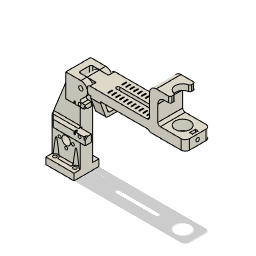
Pen-holder (Autodesk Fusion 360 design; units mm, degrees)
Autodesk Fusion 360 part; units mm, degrees
note: some values were not read from the file. Chosen so that the rebuilt part matches the saved one: which face or edge a step refers to; which pieces of a blend or face edit are solid. Set by a fixed rule: which sketch regions a step uses.
(part 1 of 2)
sketch "Sketch2" plane through (0, 0, 0) normal (0, 1, 0) x (1, 0, 0)
  circle A0 centre (1.8589, 40.0895) radius 2.1
  circle A1 centre (25.8589, 22.0895) radius 2.1
  circle A2 centre (25.8589, 40.0895) radius 2.1
  line L0 (-3.1411, 46.0895) -> (30.8589, 46.0895)
  line L1 (1.8589, 40.0895) -> (25.8589, 22.0895) construction
  line L2 (30.8589, 16.0895) -> (-3.1411, 16.0895)
  line L3 (30.8589, 46.0895) -> (30.8589, 16.0895)
  line L4 (-3.1411, 16.0895) -> (-3.1411, 46.0895)
  line L5 (25.8589, 40.0895) -> (1.8589, 22.0895) construction
  circle A3 centre (1.8589, 22.0895) radius 2.1
  point P0 (13.8589, 31.0895)
  dimension "d22" = 30
  dimension "d24" = 18
  dimension "d25" = 18
  dimension "d26" = 4.2
  dimension "d27" = 4.2
  dimension "d28" = 4.2
  dimension "d29" = 4.2
  dimension "d30" = 15
  dimension "d453" = 18
  dimension "d617" = 17
  dimension "d618" = 34
  constraint horizontal L0
  constraint vertical L3
  constraint horizontal L2
  constraint vertical L4
  constraint coincident A0.centre L1.start
  constraint coincident A1.centre L1.end
  constraint coincident A2.centre L5.start
  constraint coincident L5.end A3.centre
  constraint midpoint P0 L1
  measures "d22" distance of L0 L2
  measures "d24" distance of A2.centre A1.centre
  measures "d25" distance of L5.end A0.centre
  measures "d26" diameter of A0
  measures "d27" diameter of A2
  measures "d28" diameter of A1
  measures "d29" diameter of A3
  measures "d30" distance of P0 L2
  measures "d453" vertical distance of A1.centre A0.centre
  measures "d617" distance of P0 L3
  measures "d618" distance of L0.start L0.end
extrude "Extrude2" add sketch "Sketch2" along normal blind 8 makes body 1
sketch "Sketch3" plane through (0, 8, 0) normal (0, 1, 0) x (-1, 0, 0)
  circle A0 centre (-1.8589, -22.0895) radius 2.1
  circle A1 centre (-25.8589, -22.0895) radius 2.1
  circle A2 centre (-1.8589, -40.0895) radius 2.1
  circle A3 centre (-25.8589, -40.0895) radius 2.1
  line L0 (3.1411, -16.0895) -> (-30.8589, -16.0895)
  line L1 (-30.8589, -16.0895) -> (-30.8589, -46.0895)
  line L2 (-30.8589, -46.0895) -> (3.1411, -46.0895)
  line L3 (3.1411, -46.0895) -> (3.1411, -16.0895)
  line L4 (3.1411, -38.5895) -> (-30.8589, -38.5895)
  line L5 (-30.8589, -38.5895) -> (-30.8589, -23.5895)
  line L6 (-30.8589, -23.5895) -> (3.1411, -23.5895)
  line L7 (3.1411, -23.5895) -> (3.1411, -38.5895)
  circle A4 centre (-1.8589, -40.0895) radius 3.5
  circle A5 centre (-25.8589, -40.0895) radius 3.5
  circle A6 centre (-25.8589, -22.0895) radius 3.5
  circle A7 centre (-1.8589, -22.0895) radius 3.5
  dimension "d46" = 15
  dimension "d47" = 1.5
  dimension "d48" = 18
  dimension "d49" = 7
  dimension "d50" = 7
  dimension "d51" = 7
  dimension "d52" = 7
  constraint horizontal L4
  constraint vertical L5
  constraint horizontal L6
  constraint vertical L7
  constraint coincident L1 L5.end
  constraint coincident L3 L4.start
  constraint concentric A2 A4
  constraint concentric A3 A5
  constraint concentric A1 A6
  constraint concentric A0 A7
  measures "d46" distance of L4 L6
  measures "d47" distance of A2.centre L4
  measures "d48" distance of A0.centre A2.centre
  measures "d49" diameter of A7
  measures "d50" diameter of A6
  measures "d51" diameter of A5
  measures "d52" diameter of A4
extrude "Extrude3" add sketch "Sketch3" along normal blind 41 contours A0 L6 | A0 L6 A7 | L1 L3 L4 L5 L6 L7 A4 A5 A6 A7 | A1 L6 A6 | A1 L6 | A2 L4 A4 | A2 L4 | A3 L4 A5 | A3 L4 picked at (-2.2737, -23.6533) picked at (-1.6456, -25.1095) picked at (-26.0721, -25.1095) picked at (-26.2737, -23.6533) picked at (-2.0721, -37.0694) picked at (-1.9915, -38.2108) picked at (-25.6456, -37.0694) picked at (-25.8096, -38.3912) bodies 1
sketch "Sketch4" plane through (0, 0, -38.5895) normal (0, 0, -1) x (-1, 0, 0)
  line L0 (-0.3892, 8) -> (3.1411, 8)
  line L1 (3.1411, 8) -> (3.1411, 49)
  line L2 (3.1411, 49) -> (-30.8589, 49)
  line L3 (-30.8589, 49) -> (-30.8589, 8)
  circle A0 centre (-13.8589, 30) radius 11.1
  circle A1 centre (-13.8589, 30) radius 5.2
  line L4 (3.1411, 0) -> (-30.8589, 0)
  line L5 (-30.8589, 8) -> (-27.3286, 8)
  line L6 (-27.3286, 8) -> (-24.3892, 8)
  line L7 (-24.3892, 8) -> (-3.3286, 8)
  line L8 (-3.3286, 8) -> (-0.3892, 8)
  dimension "d40" = 10.4
  dimension "d41" = 22.2
  dimension "d66" = 30
  dimension "d619" = 34
  dimension "d620" = 17
  dimension "d621" = 17
  measures "d40" diameter of A1
  measures "d41" diameter of A0
  measures "d66" distance of A0.centre L4
  measures "d619" distance of L1.end L2.end
  measures "d620" distance of L3 A0.centre
  measures "d621" distance of L3 A0.centre
extrude "Extrude4" cut sketch "Sketch4" against normal blind 5 contours A0 bodies 1
extrude "Extrude5" cut sketch "Sketch4" against normal blind 15 contours A1 bodies 1
sketch "Sketch6" plane through (0, 0, -33.5895) normal (0, 0, -1) x (-1, 0, 0)
  circle A0 centre (-13.8589, 30) radius 5.2
  line L0 (-13.8589, 30) -> (10.0526, 30) construction
  line L1 (-13.8589, 30) -> (-13.8589, 48.2161) construction
  line L2 (-13.8589, 30) -> (-31.0155, 30) construction
  line L3 (-13.8589, 30) -> (-13.8589, 12.744) construction
  circle A1 centre (-13.8589, 30) radius 8 construction
  circle A2 centre (-13.8589, 38) radius 1.75
  circle A3 centre (-5.8589, 30) radius 1.75
  circle A4 centre (-13.8589, 22) radius 1.75
  circle A5 centre (-21.8589, 30) radius 1.75
  circle A6 centre (-13.8589, 30) radius 11.1
  dimension "d60" = 16
  dimension "d61" = 3.5
  dimension "d62" = 3.5
  dimension "d63" = 3.5
  dimension "d64" = 3.5
  constraint coincident A0.centre L0.start
  constraint horizontal L0
  constraint perpendicular L0 L1
  constraint perpendicular L1 L2
  constraint perpendicular L0 L3
  constraint coincident A1 A2.centre
  constraint coincident L1 A2.centre
  constraint coincident L0 A3.centre
  constraint coincident A1 A3.centre
  constraint coincident A1 A4.centre
  constraint coincident L3 A4.centre
  constraint coincident A1 A5.centre
  constraint coincident L2 A5.centre
  measures "d60" diameter of A1
  measures "d61" diameter of A2
  measures "d62" diameter of A5
  measures "d63" diameter of A4
  measures "d64" diameter of A3
extrude "Extrude8" cut sketch "Sketch6" against normal through all contours A2 | A3 | A4 | A5 bodies 1
sketch "Sketch7" plane through (0, 0, -38.5895) normal (0, 0, -1) x (-1, 0, 0)
  line L0 (3.1411, 8) -> (3.1411, 49)
  line L1 (3.1411, 49) -> (-30.8589, 49)
  line L2 (-30.8589, 49) -> (-30.8589, 8)
  line L3 (-30.8589, 49) -> (-20.8589, 49)
  line L4 (-20.8589, 49) -> (-20.8589, 109)
  line L5 (-20.8589, 109) -> (-30.8589, 109)
  line L6 (-30.8589, 109) -> (-30.8589, 49)
  line L7 (3.1411, 49) -> (-20.8589, 109)
  line L8 (-30.8589, 109) -> (-6.8589, 49)
  line L9 (-30.8589, 8) -> (-27.3286, 8)
  line L10 (-27.3286, 8) -> (-24.3892, 8)
  line L11 (-24.3892, 8) -> (-3.3286, 8)
  line L12 (-3.3286, 8) -> (-0.3892, 8)
  line L13 (-0.3892, 8) -> (3.1411, 8)
  circle A0 centre (-13.8589, 30) radius 11.1
  line L14 (-30.8589, 109) -> (3.1411, 109)
  line L15 (3.1411, 109) -> (3.1411, 99)
  line L16 (3.1411, 99) -> (-30.8589, 99)
  line L17 (-30.8589, 99) -> (-30.8589, 109)
  line L18 (3.1411, 49) -> (-6.8589, 49)
  line L19 (-6.8589, 49) -> (-6.8589, 109)
  line L20 (-6.8589, 109) -> (3.1411, 109)
  line L21 (3.1411, 109) -> (3.1411, 49)
  dimension "d72" = 60
  dimension "d73" = 10
  dimension "d639" = 10
  dimension "d640" = 10
  dimension "d641" = 10
  constraint horizontal L3
  constraint vertical L4
  constraint horizontal L5
  constraint vertical L6
  constraint coincident L1.end L2.start
  constraint coincident L0.end L1.start
  constraint coincident L1 L8.end
  constraint parallel L7 L8
  constraint horizontal L14
  constraint vertical L15
  constraint horizontal L16
  constraint vertical L17
  constraint horizontal L18
  constraint vertical L19
  constraint horizontal L20
  constraint vertical L21
  constraint coincident L14 L19.end
  measures "d72" distance of L3 L5
  measures "d73" distance of L4 L6
  measures "d639" distance of L19 L21
  measures "d640" distance of L14.end L15.end
  measures "d641" distance of L14.end L19
extrude "Extrude9" add sketch "Sketch7" against normal up to surface (15 mm away) contours L1 L7 L18 L19 | L1 L4 L8 | L4 L7 L8 L16 L19 | L1 L3 L4 L6 L8 L16 | L4 L8 L16 | L4 L7 L16 | L4 L5 L8 L14 L16 | L6 L8 L16 L17 bodies 1
sketch "Sketch8" plane through (0, 0, -23.5895) normal (0, 0, 1) x (1, 0, 0)
  line L0 (-3.1411, 49) -> (-3.1411, 8)
  line L1 (30.8589, 8) -> (30.8589, 109)
  line L2 (30.8589, 109) -> (20.8589, 109)
  circle A0 centre (5.8589, 30) radius 1.75
  circle A1 centre (13.8589, 22) radius 1.75
  line L3 (30.8589, 85.9) -> (44.3589, 85.9)
  line L4 (44.3589, 85.9) -> (44.3589, 80.9)
  line L5 (44.3589, 80.9) -> (30.8589, 80.9)
  line L6 (30.8589, 80.9) -> (30.8589, 85.9)
  line L7 (30.8589, 46.9) -> (44.3589, 46.9)
  line L8 (44.3589, 46.9) -> (44.3589, 51.9)
  line L9 (44.3589, 51.9) -> (30.8589, 51.9)
  line L10 (30.8589, 51.9) -> (30.8589, 46.9)
  circle A2 centre (39.1589, 100.9) radius 8.1
  circle A3 centre (39.1589, 100.9) radius 5.1
  line L11 (39.1589, 100.9) -> (39.1589, 102.6668) construction
  line L12 (39.1589, 100.9) -> (39.1589, 81) construction
  line L13 (39.1589, 109) -> (30.8589, 109)
  line L14 (39.1589, 92.8) -> (30.8589, 92.8)
  line L15 (39.1589, 100.9) -> (49.3712, 90.6877) construction
  line L16 (39.1589, 100.9) -> (45.8085, 100.9) construction
  line L17 (44.8864, 95.1724) -> (30.8589, 81.1449)
  circle A4 centre (37.6089, 49.4) radius 1.75
  circle A5 centre (37.6089, 83.4) radius 1.75
  circle A6 centre (39.1589, 100.9) radius 2.6
  line L18 (20.8589, 109) -> (30.8589, 109)
  line L19 (30.8589, 109) -> (30.8589, 81.1449)
  line L20 (30.8589, 81.1449) -> (20.8589, 81.1449)
  line L21 (20.8589, 81.1449) -> (20.8589, 109)
  line L22 (30.8589, 46.9) -> (20.8589, 46.9)
  line L23 (20.8589, 46.9) -> (20.8589, 51.9)
  line L24 (20.8589, 51.9) -> (30.8589, 51.9)
  line L25 (30.8589, 51.9) -> (30.8589, 46.9)
  line L26 (30.8589, 85.9) -> (20.8589, 85.9)
  line L27 (20.8589, 85.9) -> (20.8589, 80.9)
  line L28 (20.8589, 80.9) -> (30.8589, 80.9)
  line L29 (30.8589, 80.9) -> (30.8589, 85.9)
  line L30 (20.8589, 46.9) -> (44.3589, 46.9)
  line L31 (44.3589, 46.9) -> (44.3589, 51.6551)
  line L32 (44.3589, 51.6551) -> (20.8589, 51.6551)
  line L33 (20.8589, 51.6551) -> (20.8589, 46.9)
  line L34 (44.3589, 85.9) -> (20.8589, 85.9)
  line L35 (20.8589, 85.9) -> (20.8589, 81.1449)
  line L36 (20.8589, 81.1449) -> (44.3589, 81.1449)
  line L37 (44.3589, 81.1449) -> (44.3589, 85.9)
  line L38 (-3.1411, 8) -> (0.3892, 8)
  circle A7 centre (13.8589, 38) radius 1.75
  circle A8 centre (21.8589, 30) radius 1.75
  circle A9 centre (13.8589, 30) radius 5.2
  line L39 (0.3892, 8) -> (3.3286, 8)
  line L40 (3.3286, 8) -> (24.3892, 8)
  line L41 (24.3892, 8) -> (27.3286, 8)
  line L42 (27.3286, 8) -> (30.8589, 8)
  line L43 (20.8589, 109) -> (19.6589, 109)
  line L44 (19.6589, 109) -> (19.6589, 81)
  line L45 (19.6589, 81) -> (20.8589, 81)
  line L46 (20.8589, 81) -> (20.8589, 109)
  line L47 (20.8589, 51.9) -> (5.8589, 51.9)
  line L48 (5.8589, 51.9) -> (5.8589, 46.9)
  line L49 (5.8589, 46.9) -> (20.8589, 46.9)
  line L50 (20.8589, 46.9) -> (20.8589, 51.9)
  line L51 (5.8589, 46.9) -> (44.3589, 46.9)
  line L52 (44.3589, 46.9) -> (44.3589, 43.4)
  line L53 (44.3589, 43.4) -> (5.8589, 43.4)
  line L54 (5.8589, 43.4) -> (5.8589, 46.9)
  line L55 (20.8589, 109) -> (-3.1411, 49)
  dimension "d76" = 29
  dimension "d77" = 13.5
  dimension "d78" = 13.5
  dimension "d79" = 5
  dimension "d80" = 5
  dimension "d81" = 10.2
  dimension "d84" = 16.2
  dimension "d85" = 16.2
  dimension "d86" = 8.3
  dimension "d87" = 45
  dimension "d90" = 3.5
  dimension "d91" = 3.5
  dimension "d92" = 2.5
  dimension "d93" = 2.5
  dimension "d94" = 6.75
  dimension "d95" = 6.75
  dimension "d100" = 5.2
  dimension "d101" = 15
  dimension "d117" = 5
  dimension "d118" = 5
  dimension "d119" = 10
  dimension "d121" = 10
  dimension "d124" = 23.5
  dimension "d125" = -4.7551
  dimension "d126" = -4.7551
  dimension "d642" = 10
  dimension "d643" = 23.1
  dimension "d644" = 23.1
  dimension "d646" = 5
  dimension "d662" = 3.5
  constraint horizontal L3
  constraint vertical L4
  constraint horizontal L5
  constraint vertical L6
  constraint coincident L1 L3.start
  constraint horizontal L7
  constraint vertical L8
  constraint horizontal L9
  constraint vertical L10
  constraint coincident L1 L7.start
  constraint concentric A2 A3
  constraint coincident A2.centre A3.centre
  constraint vertical L11
  constraint parallel L11 L12
  constraint coincident A2 L13.start
  constraint coincident L11 L13.start
  constraint coincident L1 L2.start
  constraint tangent A2 L13
  constraint coincident A2 L14.start
  constraint coincident L12 L14.start
  constraint coincident L1 L14.end
  constraint tangent A2 L14
  constraint horizontal L16
  constraint coincident L15 L17.start
  constraint coincident A2 L17.start
  constraint coincident L1 L17.end
  constraint tangent A2 L17
  constraint concentric A2 A6
  constraint horizontal L18
  constraint vertical L19
  constraint horizontal L20
  constraint vertical L21
  constraint horizontal L22
  constraint vertical L23
  constraint horizontal L24
  constraint vertical L25
  constraint horizontal L26
  constraint vertical L27
  constraint horizontal L28
  constraint vertical L29
  constraint horizontal L30
  constraint vertical L31
  constraint horizontal L32
  constraint vertical L33
  constraint horizontal L34
  constraint vertical L35
  constraint horizontal L36
  constraint vertical L37
  constraint horizontal L43
  constraint vertical L44
  constraint horizontal L45
  constraint vertical L46
  constraint horizontal L47
  constraint vertical L48
  constraint horizontal L49
  constraint vertical L50
  constraint horizontal L51
  constraint vertical L52
  constraint horizontal L53
  constraint vertical L54
  measures "d76" distance of L5 L9
  measures "d77" distance of L3.start L4
  measures "d78" distance of L8.end L9.end
  measures "d79" distance of L3.end L4.end
  measures "d80" distance of L7.end L8.end
  measures "d81" diameter of A3
  measures "d84" diameter of A2
  measures "d85" distance of L1.end L14
  measures "d86" distance of L1 A2.centre
  measures "d87" angle of L15 L16
  measures "d90" diameter of A4
  measures "d91" diameter of A5
  measures "d92" distance of L3 A5.centre
  measures "d93" distance of L9 A4.centre
  measures "d94" distance of L8 A4.centre
  measures "d95" distance of L4 A5.centre
  measures "d100" diameter of A6
  measures "d101" distance of L3 A2.centre
  measures "d117" distance of L22.end L23.end
  measures "d118" distance of L26.end L27.end
  measures "d119" distance of L27.end L5.end
  measures "d121" distance of L23.end L9.end
  measures "d124" distance of L31.end L32.end
  measures "d125" distance of L3.end L36.end
  measures "d126" distance of L7.end L31.end
  measures "d642" distance of L1.end L2.end
  measures "d643" distance of L2 L26.end
  measures "d644" distance of L18 L34
  measures "d646" distance of L47 L49
  measures "d662" distance of L7.end L52.end
extrude "Extrude12" add sketch "Sketch8" along normal blind 4.2 contours L1 L2 L18 L19 L21 L26 L34 L46 | L1 L6 L20 L27 L28 L29 L36 L46 | L1 A2 L13 L14 L19 | L1 L6 L19 L20 L21 L26 L27 L29 L34 L35 L36 L46 | L1 L3 A2 L14 L17 L19 L34 | A2 | L1 L3 L6 L17 L19 L29 L34 bodies 1
extrude "Extrude13" add sketch "Sketch8" along normal up to surface (3.3 mm away) from surface at 4.2 contours L1 L2 L18 L19 L21 L26 L34 L46 | L1 L6 L20 L27 L28 L29 L36 L46 | L1 A2 L13 L14 L19 | L1 L6 L19 L20 L21 L26 L27 L29 L34 L35 L36 L46 | L1 L3 A2 L14 L17 L19 L34 | A2 | L1 L3 L6 L17 L19 L29 L34 | A3 bodies 1
extrude "Extrude15" add sketch "Sketch8" against normal blind 3.8 from surface at -15 contours L1 L2 L18 L19 L21 L26 L34 L46 | L1 L6 L20 L27 L28 L29 L36 L46 | L1 A2 L13 L14 L19 | L1 L6 L19 L20 L21 L26 L27 L29 L34 L35 L36 L46 | L1 L3 A2 L14 L17 L19 L34 | A2 | L1 L3 L6 L17 L19 L29 L34 bodies 1
extrude "Extrude16" add sketch "Sketch8" against normal up to surface (3.7 mm away) from surface at -18.8 contours L1 L2 L18 L19 L21 L26 L34 L46 | L1 L6 L20 L27 L28 L29 L36 L46 | L1 A2 L13 L14 L19 | L1 L6 L19 L20 L21 L26 L27 L29 L34 L35 L36 L46 | L1 L3 A2 L14 L17 L19 L34 | A2 | L1 L3 L6 L17 L19 L29 L34 | A3 bodies 1
extrude "Extrude18" add sketch "Sketch8" along normal up to surface (7.5 mm away) contours L1 L6 L20 L27 L28 L29 L36 L46 | L1 L6 L19 L20 L21 L26 L27 L29 L34 L35 L36 L46 | L1 L3 L6 L17 L19 L29 L34 | L1 L4 L5 L6 L29 L36 | L3 L4 L17 L34 L36 L37 | L1 L8 L9 L10 L25 L32 | L1 L10 L23 L24 L25 L32 L50 | L1 L22 L30 L49 L51 L53 L54 | L1 L7 L30 L51 L52 L53 | L1 L7 L8 L10 L25 L30 L31 L32 L51 | L1 L10 L22 L23 L25 L30 L32 L33 L50 L51 | L23 L33 L47 L48 L49 L50 L51 bodies 1
sketch "Sketch10" plane through (44.3589, 0, 0) normal (1, 0, 0) x (0, 0, -1)
  line L0 (23.5895, 80.9) -> (23.5895, 85.9)
  line L1 (16.0895, 85.9) -> (16.0895, 80.9)
  line L2 (16.0895, 80.9) -> (23.5895, 80.9)
  line L3 (16.0895, 83.9) -> (19.0895, 80.9)
  line L4 (16.0895, 83.9) -> (35.1836, 83.9) construction
  line L5 (19.0895, 51.9) -> (16.0895, 48.9)
  line L6 (19.0895, 51.9) -> (44.7305, 51.9) construction
  line L7 (16.0895, 48.9) -> (16.0895, 51.9)
  line L8 (16.0895, 51.9) -> (19.0895, 51.9)
  line L9 (16.0895, 83.9) -> (16.0895, 80.9)
  line L10 (16.0895, 80.9) -> (19.0895, 80.9)
  line L11 (23.5895, 85.9) -> (16.0895, 85.9)
  point P0 (16.0895, 51.9)
  point P1 (23.5895, 43.4)
  point P2 (16.0895, 43.4)
  dimension "d128" = 45
  dimension "d129" = 135
  dimension "d130" = 3
  dimension "d131" = 3
  dimension "d133" = 3
  dimension "d134" = 3
  dimension "d461" = 7.5
  dimension "d462" = 7.5
  dimension "d663" = 7.5
  dimension "d664" = 7.5
  constraint horizontal L4
  constraint horizontal L6
  constraint vertical L7
  constraint perpendicular L7 L8
  constraint perpendicular L4 L9
  constraint perpendicular L9 L10
  measures "d128" angle of L3 L4
  measures "d129" angle of L5 L6
  measures "d130" distance of L3.end L1.end
  measures "d131" distance of L2 L3.start
  measures "d133" distance of L5.start P0
  measures "d134" vertical distance of L5.end P0
  measures "d461" distance of L0.start L1.end
  measures "d462" distance of L0.start L9
  measures "d663" distance of P1 P2
  measures "d664" distance of L7 P1
extrude "Extrude19" cut sketch "Sketch10" against normal blind 1.5 contours L1 L2 L3 L9 L10 | L5 L7 L8 bodies 1
extrude "Extrude20" cut sketch "Sketch10" along normal blind 1.5 from surface at -13.5 contours L1 L2 L3 L9 L10 | L5 L7 L8 bodies 1
sketch "Sketch31" plane through (0, 109, 0) normal (0, 1, 0) x (-1, 0, 0)
  line L0 (-20.8589, -16.0895) -> (-39.1589, -16.0895)
  line L1 (-39.1589, -16.0895) -> (-39.1589, -23.5895)
  line L2 (-39.1589, -23.5895) -> (-30.8589, -23.5895)
  line L3 (-30.8589, -23.5895) -> (-30.8589, -38.5895)
  line L4 (-30.8589, -38.5895) -> (-39.1589, -38.5895)
  line L5 (-39.1589, -38.5895) -> (-39.1589, -46.0895)
  line L6 (-39.1589, -46.0895) -> (-20.8589, -46.0895)
  line L7 (-28.8589, -38.6895) -> (-55.9589, -38.6895)
  line L8 (-55.9589, -38.6895) -> (-55.9589, -23.4895)
  line L9 (-55.9589, -23.4895) -> (-28.8589, -23.4895)
  line L10 (-28.8589, -23.4895) -> (-28.8589, -38.6895)
  line L11 (-20.8589, -38.5895) -> (-20.8589, -23.5895)
  line L12 (-20.8589, -23.5895) -> (-20.8589, -16.0895)
  line L13 (-20.8589, -46.0895) -> (-20.8589, -38.5895)
  dimension "d670" = 15
  dimension "d671" = 15.2
  dimension "d672" = 0.1
  dimension "d689" = 8.3
  dimension "d690" = 10.3
  constraint horizontal L7
  constraint vertical L8
  constraint horizontal L9
  constraint vertical L10
  measures "d670" distance of L2 L4
  measures "d671" distance of L7.end L8.end
  measures "d672" distance of L4 L7
  measures "d689" distance of L3.end L4.end
  measures "d690" horizontal distance of L4.end L7.start
extrude "Extrude38" cut sketch "Sketch31" against normal up to surface (23.1 mm away) contours L1 L2 L3 L4 L5 L7 L9 L10 | L1 L2 L3 L4 L5 L7 L8 L9 bodies 1
chamfer "Chamfer3" distance 7.5 angle 45 3 edges at (20.8589, 94.95, -38.5895) (20.8589, 94.95, -23.5895) (5.8589, 47.65, -23.5895) on bodies 1
fillet "Fillet27" radius 2 6 edges at (22.1089, 80.9, -23.5895) (14.6089, 43.4, -23.5895) (14.6089, 51.9, -23.5895) (22.1089, 80.9, -38.5895) (13.8589, 8, -38.5895) (13.8589, 8, -23.5895) on bodies 1
fillet "Fillet28" radius 2 5 edges at (28.8589, 97.45, -38.6895) (30.8589, 83.5224, -38.5895) (30.8589, 83.4, -23.5895) (28.8589, 97.45, -23.4895) (30.8589, 47.65, -23.5895) on bodies 1
fillet "Fillet29" radius 2 1 edges at (35.614, 85.9, -19.7895) on bodies 1
sketch "Sketch30" plane through (0, 8, 0) normal (0, 1, 0) x (-1, 0, 0)
  arc A0 (-3.8985, -40.5895) -> (-0.3892, -38.5895) centre (-1.8589, -40.0895) ccw
  arc A1 (-27.3286, -38.5895) -> (-23.8193, -40.5895) centre (-25.8589, -40.0895) ccw
  circle A2 centre (-1.8589, -40.0895) radius 4
  arc A3 (-0.3892, -23.5895) -> (-3.8985, -21.5895) centre (-1.8589, -22.0895) ccw
  arc A4 (-23.8193, -21.5895) -> (-27.3286, -23.5895) centre (-25.8589, -22.0895) ccw
  arc A5 (-27.3286, -38.5895) -> (-23.8193, -40.5895) centre (-25.8589, -40.0895) ccw
  circle A6 centre (-1.8589, -22.0895) radius 4
  circle A7 centre (-25.8589, -22.0895) radius 4
  circle A8 centre (-25.8589, -40.0895) radius 4
  line L0 (-27.3286, -38.5895) -> (-30.8589, -38.5895)
  line L1 (-30.8589, -38.5895) -> (-30.8589, -46.0895)
  line L2 (-30.8589, -46.0895) -> (3.1411, -46.0895)
  line L3 (3.1411, -46.0895) -> (3.1411, -38.5895)
  line L4 (3.1411, -38.5895) -> (-0.3892, -38.5895)
  line L5 (-3.8985, -40.5895) -> (-23.8193, -40.5895)
  dimension "d622" = 8
  dimension "d623" = 8
  dimension "d624" = 8
  dimension "d625" = 8
  constraint concentric A0 A2
  constraint concentric A3 A6
  constraint concentric A4 A7
  constraint concentric A5 A8
  measures "d622" diameter of A2
  measures "d623" diameter of A6
  measures "d624" diameter of A8
  measures "d625" diameter of A7
extrude "Extrude37" cut sketch "Sketch30" along normal through all draft -7 contours A0 A2 L4 L5 | A0 A2 L4 L5 | A1 A5 A8 L0 L5 | A1 A5 A8 L0 L5 | A6 | A7 bodies 1
sketch "Sketch12" plane through (0, 0, 0) normal (0, 1, 0) x (1, 0, 0)
  circle A0 centre (2.1847, 145.5) radius 9
  line L0 (20.3847, 160.5) -> (-12.8153, 160.5)
  line L1 (-12.8153, 160.5) -> (-12.8153, 130.5)
  line L2 (-12.8153, 130.5) -> (20.3847, 130.5)
  line L3 (20.3847, 130.5) -> (20.3847, 160.5)
  line L4 (14.1847, 142) -> (17.3847, 142)
  line L5 (17.3847, 142) -> (17.3847, 149)
  line L6 (17.3847, 149) -> (14.1847, 149)
  line L7 (14.1847, 149) -> (14.1847, 142)
  line L8 (-12.8153, 160.5) -> (-22.8153, 160.5)
  line L9 (-22.8153, 160.5) -> (-22.8153, 130.5)
  line L10 (-22.8153, 130.5) -> (-12.8153, 130.5)
  line L11 (-12.8153, 130.5) -> (-12.8153, 160.5)
  line L12 (2.1847, 145.5) -> (2.1847, 130.5)
  line L13 (2.1847, 145.5) -> (2.1847, 160.5)
  point P0 (39.1589, 46.0895)
  point P1 (39.1589, 16.0895)
  point P2 (20.8589, 16.0895)
  point P3 (20.8589, 46.0895)
  dimension "d168" = 18
  dimension "d169" = 7
  dimension "d170" = 3.2
  dimension "d171" = 3.5
  dimension "d172" = 12
  dimension "d173" = 3
  dimension "d175" = 30
  dimension "d176" = 15
  dimension "d177" = 15
  dimension "d180" = 10
  dimension "d181" = 30
  dimension "d681" = 30
  constraint horizontal L0
  constraint vertical L1
  constraint horizontal L2
  constraint vertical L3
  constraint horizontal L4
  constraint vertical L5
  constraint horizontal L6
  constraint vertical L7
  constraint horizontal L8
  constraint vertical L9
  constraint horizontal L10
  constraint vertical L11
  constraint coincident A0.centre L12.start
  constraint coincident L2 L12.end
  constraint perpendicular L2 L12
  constraint perpendicular L0 L13
  constraint coincident L0 L13.end
  measures "d168" diameter of A0
  measures "d169" distance of L4.start L6.end
  measures "d170" distance of L5.end L6.end
  measures "d171" distance of A0.centre L4
  measures "d172" distance of A0.centre L7
  measures "d173" distance of L3 L5
  measures "d175" distance of L0.start L2.end
  measures "d176" distance of A0.centre L0
  measures "d177" distance of A0.centre L1
  measures "d180" distance of L9.end L1.end
  measures "d181" distance of L0 L10
  measures "d681" distance of P0 P1
extrude "Extrude21" add sketch "Sketch12" along normal blind 12 separate body contours A0 L0 L2 L3 L12 L13 | A0 L0 L1 L2 L11 L12 L13 | L1 L8 L9 L10 L11 makes body 2
sketch "Sketch13" plane through (0, 12, 0) normal (0, 1, 0) x (-1, 0, 0)
  line L0 (-2.1847, -160.5) -> (22.8153, -160.5)
  line L1 (22.8153, -160.5) -> (22.8153, -130.5)
  line L2 (22.8153, -130.5) -> (-2.1847, -130.5)
  line L3 (22.8153, -160.5) -> (97.8153, -160.5)
  line L4 (97.8153, -160.5) -> (97.8153, -130.5)
  line L5 (97.8153, -130.5) -> (22.8153, -130.5)
  line L6 (22.8153, -130.5) -> (22.8153, -160.5)
  line L7 (77.8153, -143.5) -> (26.8153, -143.5)
  line L8 (26.8153, -143.5) -> (26.8153, -147.5)
  line L9 (26.8153, -147.5) -> (77.8153, -147.5)
  line L10 (77.8153, -147.5) -> (77.8153, -143.5)
  arc A0 (-2.1847, -154.5) -> (-2.1847, -136.5) centre (-2.1847, -145.5) ccw
  line L11 (-2.1847, -154.5) -> (-2.1847, -160.5)
  line L12 (-2.1847, -130.5) -> (-2.1847, -136.5)
  circle A1 centre (-2.1847, -145.5) radius 9
  line L13 (-14.1847, -142) -> (-14.1847, -149)
  line L14 (-14.1847, -149) -> (-17.3847, -149)
  line L15 (-17.3847, -149) -> (-17.3847, -142)
  line L16 (-17.3847, -142) -> (-14.1847, -142)
  line L17 (-20.3847, -130.5) -> (-20.3847, -160.5)
  line L18 (-20.3847, -160.5) -> (22.8153, -160.5)
  line L19 (22.8153, -130.5) -> (-20.3847, -130.5)
  line L20 (22.8153, -160.5) -> (22.8153, -130.5)
  point P0 (12.8153, -160.5)
  point P1 (12.8153, -130.5)
  point P2 (-2.1847, -145.5)
  dimension "d187" = 30
  dimension "d188" = 30
  dimension "d189" = 100
  dimension "d190" = 4
  dimension "d191" = 13
  dimension "d192" = 20
  dimension "d193" = 4
  constraint horizontal L3
  constraint vertical L4
  constraint horizontal L5
  constraint vertical L6
  constraint coincident L0.end L1.start
  constraint horizontal L7
  constraint vertical L8
  constraint horizontal L9
  constraint vertical L10
  measures "d187" distance of P0 P1
  measures "d188" distance of L3.end L4.end
  measures "d189" distance of L4 P2
  measures "d190" distance of L7 L9
  measures "d191" distance of L3 L9
  measures "d192" distance of L4 L10
  measures "d193" distance of L6 L8.end
extrude "Extrude24" add sketch "Sketch13" against normal blind 10 contours L1 L3 L4 L5 L6 L20 bodies 2
sketch "Sketch14" plane through (0, 0, -160.5) normal (0, 0, -1) x (-1, 0, 0)
  line L0 (-20.3847, 0) -> (22.8153, 0)
  line L1 (97.8153, 2) -> (97.8153, 12)
  line L2 (97.8153, 12) -> (-20.3847, 12)
  line L3 (-20.3847, 12) -> (-20.3847, 0)
  circle A0 centre (105.8153, 4) radius 2.5
  circle A1 centre (105.8153, 4) radius 8
  line L4 (97.8153, 12) -> (105.8153, 12)
  line L5 (97.8153, 2) -> (98.7565, 0.2353)
  line L6 (97.8153, 12) -> (97.8153, 2)
  line L7 (22.8153, 0) -> (22.8153, 2)
  line L8 (22.8153, 2) -> (97.8153, 2)
  dimension "d196" = 5
  dimension "d197" = 16
  dimension "d198" = 8
  dimension "d199" = 8
  constraint concentric A0 A1
  constraint coincident L1.end L2.start
  constraint perpendicular L1 L4
  constraint coincident L1.start L5.start
  constraint coincident A1 L5.end
  constraint tangent A1 L5
  constraint coincident A1 L4.end
  measures "d196" diameter of A0
  measures "d197" diameter of A1
  measures "d198" vertical distance of L1.end A0.centre
  measures "d199" horizontal distance of L1.end A0.centre
extrude "Extrude25" add sketch "Sketch14" against normal up to surface (30 mm away) contours L1 A1 L4 L6 | L1 A1 L5 L6 | A1 bodies 2
sketch "Sketch15" plane through (20.3847, 0, 0) normal (-1, 0, 0) x (0, 0, 1)
  line L0 (-130.5, 2) -> (-160.5, 2)
  line L1 (-160.5, 2) -> (-160.5, 0)
  line L2 (-160.5, 0) -> (-130.5, 0)
  line L3 (-130.5, 0) -> (-130.5, 2)
  line L4 (-147.5, 0) -> (-143.5, 0)
  line L5 (-143.5, 0) -> (-147.5, 0)
  line L6 (-160.5, 0) -> (-153.9485, -18)
  line L7 (-153.9485, -18) -> (-137.0515, -18)
  line L8 (-137.0515, -18) -> (-130.5, 0)
  line L9 (-156.9712, 2) -> (-151.1477, -14)
  line L10 (-151.1477, -14) -> (-139.8523, -14)
  line L11 (-139.8523, -14) -> (-134.0288, 2)
  line L12 (-160.5, -0.5) -> (-160.5, 4.5)
  line L13 (-130.5, -0.5) -> (-130.5, 4.5)
  line L14 (-160.5, -0.5) -> (-160.5, 4.5)
  line L15 (-130.5, 2) -> (-176.6254, 2) construction
  line L16 (-154.5, 0) -> (-136.5, 0)
  line L17 (-149, 0) -> (-142, 0)
  line L18 (-142, 0) -> (-149, 0)
  line L19 (-160.5, 0) -> (-130.5, 0)
  line L20 (-130.5, 0) -> (-160.5, 0)
  line L21 (-130.5, 0) -> (-160.5, 0)
  line L22 (-160.5, 0) -> (-160.5, 12)
  line L23 (-160.5, 12) -> (-130.5, 12)
  line L24 (-130.5, 12) -> (-130.5, 0)
  point P0 (-130.5, 0)
  dimension "d202" = 4
  dimension "d203" = 4
  dimension "d204" = 4
  dimension "d205" = 110
  dimension "d206" = 110
  dimension "d208" = 20
  constraint coincident L1.end L2.start
  constraint perpendicular L1 L7
  constraint coincident P0 L2.end
  constraint horizontal L10
  constraint parallel L8 L11
  constraint parallel L6 L9
  constraint coincident L0 L9.start
  constraint coincident L0 L11.end
  constraint midpoint L13 L0.start
  constraint perpendicular L13 L15
  measures "d202" distance of L7 L10
  measures "d203" distance of L8 L11
  measures "d204" distance of L6 L9
  measures "d205" angle of L6 L7
  measures "d206" angle of L7 L8
  measures "d208" distance of L7 L15
extrude "Extrude26" add sketch "Sketch15" against normal blind 12 from surface at 114.2 contours L0 L2 L3 L11 L13 L19 L20 L21 L24 | L2 L6 L7 L8 L9 L10 L11 L19 L20 L21 | L0 L1 L2 L9 L12 L14 L19 L20 L21 L22 bodies 2
sketch "Sketch16" plane through (0, 12, 0) normal (0, 1, 0) x (-1, 0, 0)
  line L0 (-20.3847, -160.5) -> (105.8153, -160.5)
  line L1 (105.8153, -130.5) -> (-20.3847, -130.5)
  line L2 (29.1937, -139.5) -> (30.1937, -139.5)
  line L3 (30.1937, -139.5) -> (30.1937, -134.5)
  line L4 (30.1937, -134.5) -> (29.1937, -134.5)
  line L5 (29.1937, -134.5) -> (29.1937, -139.5)
  line L6 (26.8153, -147.5) -> (26.8153, -143.5)
  line L7 (77.8153, -143.5) -> (77.8153, -147.5)
  line L8 (26.8153, -143.5) -> (77.8153, -143.5)
  line L9 (34.8937, -134.5) -> (33.8937, -134.5)
  line L10 (33.8937, -139.5) -> (34.8937, -139.5)
  line L11 (34.8937, -139.5) -> (34.8937, -134.5)
  line L12 (33.8937, -134.5) -> (33.8937, -139.5)
  line L13 (39.5937, -134.5) -> (38.5937, -134.5)
  line L14 (38.5937, -139.5) -> (39.5937, -139.5)
  line L15 (39.5937, -139.5) -> (39.5937, -134.5)
  line L16 (38.5937, -134.5) -> (38.5937, -139.5)
  line L17 (44.2937, -134.5) -> (43.2937, -134.5)
  line L18 (43.2937, -139.5) -> (44.2937, -139.5)
  line L19 (44.2937, -139.5) -> (44.2937, -134.5)
  line L20 (43.2937, -134.5) -> (43.2937, -139.5)
  line L21 (48.9937, -134.5) -> (47.9937, -134.5)
  line L22 (47.9937, -139.5) -> (48.9937, -139.5)
  line L23 (48.9937, -139.5) -> (48.9937, -134.5)
  line L24 (47.9937, -134.5) -> (47.9937, -139.5)
  line L25 (53.6937, -134.5) -> (52.6937, -134.5)
  line L26 (52.6937, -139.5) -> (53.6937, -139.5)
  line L27 (53.6937, -139.5) -> (53.6937, -134.5)
  line L28 (52.6937, -134.5) -> (52.6937, -139.5)
  line L29 (58.3937, -134.5) -> (57.3937, -134.5)
  line L30 (57.3937, -139.5) -> (58.3937, -139.5)
  line L31 (58.3937, -139.5) -> (58.3937, -134.5)
  line L32 (57.3937, -134.5) -> (57.3937, -139.5)
  line L33 (63.0937, -134.5) -> (62.0937, -134.5)
  line L34 (62.0937, -139.5) -> (63.0937, -139.5)
  line L35 (63.0937, -139.5) -> (63.0937, -134.5)
  line L36 (62.0937, -134.5) -> (62.0937, -139.5)
  line L37 (67.7937, -134.5) -> (66.7937, -134.5)
  line L38 (66.7937, -139.5) -> (67.7937, -139.5)
  line L39 (67.7937, -139.5) -> (67.7937, -134.5)
  line L40 (66.7937, -134.5) -> (66.7937, -139.5)
  line L41 (72.4937, -134.5) -> (71.4937, -134.5)
  line L42 (71.4937, -139.5) -> (72.4937, -139.5)
  line L43 (72.4937, -139.5) -> (72.4937, -134.5)
  line L44 (71.4937, -134.5) -> (71.4937, -139.5)
  line L45 (77.1937, -134.5) -> (76.1937, -134.5)
  line L46 (76.1937, -139.5) -> (77.1937, -139.5)
  line L47 (77.1937, -139.5) -> (77.1937, -134.5)
  line L48 (76.1937, -134.5) -> (76.1937, -139.5)
  line L49 (77.8153, -145.5) -> (26.8153, -145.5) construction
  line L50 (67.7937, -156.5) -> (66.7937, -156.5)
  line L51 (47.9937, -151.5) -> (48.9937, -151.5)
  line L52 (71.4937, -156.5) -> (71.4937, -151.5)
  line L53 (63.0937, -156.5) -> (62.0937, -156.5)
  line L54 (44.2937, -156.5) -> (43.2937, -156.5)
  line L55 (38.5937, -156.5) -> (38.5937, -151.5)
  line L56 (76.1937, -151.5) -> (77.1937, -151.5)
  line L57 (48.9937, -156.5) -> (47.9937, -156.5)
  line L58 (44.2937, -151.5) -> (44.2937, -156.5)
  line L59 (38.5937, -151.5) -> (39.5937, -151.5)
  line L60 (39.5937, -151.5) -> (39.5937, -156.5)
  line L61 (48.9937, -151.5) -> (48.9937, -156.5)
  line L62 (43.2937, -156.5) -> (43.2937, -151.5)
  line L63 (66.7937, -151.5) -> (67.7937, -151.5)
  line L64 (53.6937, -151.5) -> (53.6937, -156.5)
  line L65 (43.2937, -151.5) -> (44.2937, -151.5)
  line L66 (52.6937, -156.5) -> (52.6937, -151.5)
  line L67 (76.1937, -156.5) -> (76.1937, -151.5)
  line L68 (30.1937, -151.5) -> (30.1937, -156.5)
  line L69 (29.1937, -156.5) -> (29.1937, -151.5)
  line L70 (62.0937, -156.5) -> (62.0937, -151.5)
  line L71 (67.7937, -151.5) -> (67.7937, -156.5)
  line L72 (34.8937, -151.5) -> (34.8937, -156.5)
  line L73 (71.4937, -151.5) -> (72.4937, -151.5)
  line L74 (53.6937, -156.5) -> (52.6937, -156.5)
  line L75 (72.4937, -156.5) -> (71.4937, -156.5)
  line L76 (29.1937, -151.5) -> (30.1937, -151.5)
  line L77 (57.3937, -151.5) -> (58.3937, -151.5)
  line L78 (58.3937, -151.5) -> (58.3937, -156.5)
  line L79 (66.7937, -156.5) -> (66.7937, -151.5)
  line L80 (47.9937, -156.5) -> (47.9937, -151.5)
  line L81 (58.3937, -156.5) -> (57.3937, -156.5)
  line L82 (30.1937, -156.5) -> (29.1937, -156.5)
  line L83 (77.1937, -156.5) -> (76.1937, -156.5)
  line L84 (52.6937, -151.5) -> (53.6937, -151.5)
  line L85 (33.8937, -156.5) -> (33.8937, -151.5)
  line L86 (57.3937, -156.5) -> (57.3937, -151.5)
  line L87 (33.8937, -151.5) -> (34.8937, -151.5)
  line L88 (34.8937, -156.5) -> (33.8937, -156.5)
  line L89 (63.0937, -151.5) -> (63.0937, -156.5)
  line L90 (39.5937, -156.5) -> (38.5937, -156.5)
  line L91 (77.1937, -151.5) -> (77.1937, -156.5)
  line L92 (62.0937, -151.5) -> (63.0937, -151.5)
  line L93 (72.4937, -151.5) -> (72.4937, -156.5)
  line L94 (105.8153, -160.5) -> (105.8153, -130.5)
  circle A0 centre (-2.1847, -145.5) radius 9
  line L95 (-14.1847, -142) -> (-14.1847, -149)
  line L96 (-14.1847, -149) -> (-17.3847, -149)
  line L97 (-17.3847, -149) -> (-17.3847, -142)
  line L98 (-17.3847, -142) -> (-14.1847, -142)
  line L99 (-20.3847, -130.5) -> (-20.3847, -160.5)
  dimension "d234" = 51
  dimension "d235" = 1
  dimension "d236" = 5
  dimension "d237" = 13
  dimension "d238" = 4
  dimension "d241" = 47
  dimension "d242" = 0
  constraint horizontal L2
  constraint vertical L3
  constraint horizontal L4
  constraint vertical L5
  constraint midpoint L7 L49.start
  constraint midpoint L6 L49.end
  constraint symmetric L2.start L49 L69.end
  constraint symmetric L2.end L49 L68.start
  constraint symmetric L3.end L49 L68.end
  constraint symmetric L4.end L49 L69.start
  constraint symmetric L9.end L49 L85.start
  constraint symmetric L10.end L49 L72.start
  constraint symmetric L9.start L49 L72.end
  constraint symmetric L10.start L49 L85.end
  constraint symmetric L13.end L49 L55.start
  constraint symmetric L14.end L49 L59.end
  constraint symmetric L13.start L49 L60.end
  constraint symmetric L14.start L49 L55.end
  constraint symmetric L17.end L49 L54.end
  constraint symmetric L18.end L49 L58.start
  constraint symmetric L17.start L49 L54.start
  constraint symmetric L18.start L49 L62.end
  constraint symmetric L21.end L49 L57.end
  constraint symmetric L22.end L49 L51.end
  constraint symmetric L21.start L49 L57.start
  constraint symmetric L22.start L49 L51.start
  constraint symmetric L25.end L49 L66.start
  constraint symmetric L26.end L49 L64.start
  constraint symmetric L25.start L49 L64.end
  constraint symmetric L26.start L49 L66.end
  constraint symmetric L29.end L49 L81.end
  constraint symmetric L30.end L49 L77.end
  constraint symmetric L29.start L49 L78.end
  constraint symmetric L30.start L49 L77.start
  constraint symmetric L33.end L49 L53.end
  constraint symmetric L34.end L49 L89.start
  constraint symmetric L33.start L49 L53.start
  constraint symmetric L34.start L49 L70.end
  constraint symmetric L37.end L49 L50.end
  constraint symmetric L38.end L49 L63.end
  constraint symmetric L37.start L49 L50.start
  constraint symmetric L38.start L49 L63.start
  constraint symmetric L41.end L49 L52.start
  constraint symmetric L42.end L49 L73.end
  constraint symmetric L41.start L49 L75.start
  constraint symmetric L42.start L49 L52.end
  constraint symmetric L45.end L49 L67.start
  constraint symmetric L46.end L49 L56.end
  constraint symmetric L45.start L49 L83.start
  constraint symmetric L46.start L49 L56.start
  measures "d234" distance of L6 L7
  measures "d235" distance of L2.start L2.end
  measures "d236" distance of L2.end L3.end
  measures "d237" distance of L1 L8
  measures "d238" distance of L1 L4
extrude "Extrude27" cut sketch "Sketch16" against normal blind 1 contours L2 L3 L4 L5 | L9 L10 L11 L12 | L13 L14 L15 L16 | L17 L18 L19 L20 | L21 L22 L23 L24 | L25 L26 L27 L28 | L29 L30 L31 L32 | L33 L34 L35 L36 | L37 L38 L39 L40 | L41 L42 L43 L44 | L45 L46 L47 L48 | L50 L63 L71 L79 | L51 L57 L61 L80 | L52 L73 L75 L93 | L53 L70 L89 L92 | L54 L58 L62 L65 | L55 L59 L60 L90 | L56 L67 L83 L91 | L64 L66 L74 L84 | L68 L69 L76 L82 | L72 L85 L87 L88 | L77 L78 L81 L86 bodies 2
extrude "Extrude31" add sketch "Sketch12" along normal blind 30 from surface at 12 contours L1 L8 L9 L10 L11 bodies 2
extrude "Extrude33" add sketch "Sketch12" along normal blind 7 from surface at 42 contours A0 L0 L1 L2 L11 L12 L13 | L1 L8 L9 L10 L11 bodies 2
extrude "Extrude39" add sketch "Sketch12" along normal blind 2 contours L4 L5 L6 L7 bodies 2
sketch "Sketch28" plane through (0, 12, 0) normal (0, 1, 0) x (-1, 0, 0)
  line L0 (22.8153, -130.5) -> (22.8153, -160.5)
  line L1 (22.8153, -160.5) -> (105.8153, -160.5)
  line L2 (105.8153, -160.5) -> (105.8153, -130.5)
  line L3 (105.8153, -130.5) -> (22.8153, -130.5)
  line L4 (44.2937, -156.5) -> (43.2937, -156.5)
  line L5 (43.2937, -156.5) -> (43.2937, -151.5)
  line L6 (43.2937, -151.5) -> (44.2937, -151.5)
  line L7 (44.2937, -151.5) -> (44.2937, -156.5)
  line L8 (44.2937, -139.5) -> (43.2937, -139.5)
  line L9 (43.2937, -139.5) -> (43.2937, -134.5)
  line L10 (43.2937, -134.5) -> (44.2937, -134.5)
  line L11 (44.2937, -134.5) -> (44.2937, -139.5)
  line L12 (39.5937, -139.5) -> (38.5937, -139.5)
  line L13 (38.5937, -139.5) -> (38.5937, -134.5)
  line L14 (38.5937, -134.5) -> (39.5937, -134.5)
  line L15 (39.5937, -134.5) -> (39.5937, -139.5)
  line L16 (76.1937, -156.5) -> (76.1937, -151.5)
  line L17 (76.1937, -151.5) -> (77.1937, -151.5)
  line L18 (77.1937, -151.5) -> (77.1937, -156.5)
  line L19 (77.1937, -156.5) -> (76.1937, -156.5)
  line L20 (48.9937, -151.5) -> (48.9937, -156.5)
  line L21 (48.9937, -156.5) -> (47.9937, -156.5)
  line L22 (47.9937, -156.5) -> (47.9937, -151.5)
  line L23 (47.9937, -151.5) -> (48.9937, -151.5)
  line L24 (58.3937, -151.5) -> (58.3937, -156.5)
  line L25 (58.3937, -156.5) -> (57.3937, -156.5)
  line L26 (57.3937, -156.5) -> (57.3937, -151.5)
  line L27 (57.3937, -151.5) -> (58.3937, -151.5)
  line L28 (38.5937, -151.5) -> (39.5937, -151.5)
  line L29 (39.5937, -151.5) -> (39.5937, -156.5)
  line L30 (39.5937, -156.5) -> (38.5937, -156.5)
  line L31 (38.5937, -156.5) -> (38.5937, -151.5)
  line L32 (71.4937, -156.5) -> (71.4937, -151.5)
  line L33 (71.4937, -151.5) -> (72.4937, -151.5)
  line L34 (72.4937, -151.5) -> (72.4937, -156.5)
  line L35 (72.4937, -156.5) -> (71.4937, -156.5)
  line L36 (58.3937, -139.5) -> (57.3937, -139.5)
  line L37 (57.3937, -139.5) -> (57.3937, -134.5)
  line L38 (57.3937, -134.5) -> (58.3937, -134.5)
  line L39 (58.3937, -134.5) -> (58.3937, -139.5)
  line L40 (72.4937, -139.5) -> (71.4937, -139.5)
  line L41 (71.4937, -139.5) -> (71.4937, -134.5)
  line L42 (71.4937, -134.5) -> (72.4937, -134.5)
  line L43 (72.4937, -134.5) -> (72.4937, -139.5)
  line L44 (48.9937, -139.5) -> (47.9937, -139.5)
  line L45 (47.9937, -139.5) -> (47.9937, -134.5)
  line L46 (47.9937, -134.5) -> (48.9937, -134.5)
  line L47 (48.9937, -134.5) -> (48.9937, -139.5)
  line L48 (63.0937, -139.5) -> (62.0937, -139.5)
  line L49 (62.0937, -139.5) -> (62.0937, -134.5)
  line L50 (62.0937, -134.5) -> (63.0937, -134.5)
  line L51 (63.0937, -134.5) -> (63.0937, -139.5)
  line L52 (67.7937, -139.5) -> (66.7937, -139.5)
  line L53 (66.7937, -139.5) -> (66.7937, -134.5)
  line L54 (66.7937, -134.5) -> (67.7937, -134.5)
  line L55 (67.7937, -134.5) -> (67.7937, -139.5)
  line L56 (34.8937, -139.5) -> (33.8937, -139.5)
  line L57 (33.8937, -139.5) -> (33.8937, -134.5)
  line L58 (33.8937, -134.5) -> (34.8937, -134.5)
  line L59 (34.8937, -134.5) -> (34.8937, -139.5)
  line L60 (29.1937, -151.5) -> (30.1937, -151.5)
  line L61 (30.1937, -151.5) -> (30.1937, -156.5)
  line L62 (30.1937, -156.5) -> (29.1937, -156.5)
  line L63 (29.1937, -156.5) -> (29.1937, -151.5)
  line L64 (67.7937, -151.5) -> (67.7937, -156.5)
  line L65 (67.7937, -156.5) -> (66.7937, -156.5)
  line L66 (66.7937, -156.5) -> (66.7937, -151.5)
  line L67 (66.7937, -151.5) -> (67.7937, -151.5)
  line L68 (33.8937, -151.5) -> (34.8937, -151.5)
  line L69 (34.8937, -151.5) -> (34.8937, -156.5)
  line L70 (34.8937, -156.5) -> (33.8937, -156.5)
  line L71 (33.8937, -156.5) -> (33.8937, -151.5)
  line L72 (53.6937, -156.5) -> (52.6937, -156.5)
  line L73 (52.6937, -156.5) -> (52.6937, -151.5)
  line L74 (52.6937, -151.5) -> (53.6937, -151.5)
  line L75 (53.6937, -151.5) -> (53.6937, -156.5)
  line L76 (63.0937, -156.5) -> (62.0937, -156.5)
  line L77 (62.0937, -156.5) -> (62.0937, -151.5)
  line L78 (62.0937, -151.5) -> (63.0937, -151.5)
  line L79 (63.0937, -151.5) -> (63.0937, -156.5)
  line L80 (30.1937, -139.5) -> (29.1937, -139.5)
  line L81 (29.1937, -139.5) -> (29.1937, -134.5)
  line L82 (29.1937, -134.5) -> (30.1937, -134.5)
  line L83 (30.1937, -134.5) -> (30.1937, -139.5)
  line L84 (53.6937, -139.5) -> (52.6937, -139.5)
  line L85 (52.6937, -139.5) -> (52.6937, -134.5)
  line L86 (52.6937, -134.5) -> (53.6937, -134.5)
  line L87 (53.6937, -134.5) -> (53.6937, -139.5)
  line L88 (77.1937, -139.5) -> (76.1937, -139.5)
  line L89 (76.1937, -139.5) -> (76.1937, -134.5)
  line L90 (76.1937, -134.5) -> (77.1937, -134.5)
  line L91 (77.1937, -134.5) -> (77.1937, -139.5)
  line L92 (77.8153, -143.5) -> (77.8153, -147.5)
  line L93 (77.8153, -147.5) -> (26.8153, -147.5)
  line L94 (26.8153, -147.5) -> (26.8153, -143.5)
  line L95 (26.8153, -143.5) -> (77.8153, -143.5)
  line L96 (97.8153, -160.5) -> (127.8153, -160.5)
  line L97 (127.8153, -160.5) -> (127.8153, -153)
  line L98 (127.8153, -153) -> (97.8153, -153)
  line L99 (97.8153, -153) -> (97.8153, -160.5)
  line L100 (97.8153, -130.5) -> (127.8153, -130.5)
  line L101 (127.8153, -130.5) -> (127.8153, -138)
  line L102 (127.8153, -138) -> (97.8153, -138)
  line L103 (97.8153, -138) -> (97.8153, -130.5)
  point P0 (97.8153, -130.5)
  point P1 (97.8153, -160.5)
  point P2 (-39.1589, -38.6895)
  point P3 (-39.1589, -46.0895)
  point P4 (-39.1589, -23.4895)
  point P5 (-39.1589, -16.0895)
  dimension "d517" = 30
  dimension "d518" = 30
  dimension "d519" = 7.5
  dimension "d520" = 7.5
  dimension "d682" = 30
  dimension "d683" = 30
  dimension "d684" = 7.4
  constraint horizontal L96
  constraint vertical L97
  constraint horizontal L98
  constraint vertical L99
  constraint coincident P1 L96.start
  constraint horizontal L100
  constraint vertical L101
  constraint horizontal L102
  constraint vertical L103
  constraint coincident P0 L100.start
  measures "d517" distance of P1 L96.end
  measures "d518" distance of P0 L100.end
  measures "d519" distance of L100 L102
  measures "d520" distance of L96.end L97.end
  measures "d682" distance of L96.end L100.end
  measures "d683" distance of P3 P5
  measures "d684" distance of P4 P5
extrude "Extrude35" cut sketch "Sketch28" against normal through all contours L2 L3 L100 L102 L103 | L1 L2 L96 L98 L99 | L2 L100 L101 L102 | L2 L96 L97 L98 bodies 2
sketch "Sketch29" plane through (20.3847, 0, 0) normal (1, 0, 0) x (0, 0, -1)
  line L0 (145.5, 2) -> (145.5, 12) construction
  line L1 (149, 2) -> (149, 12) construction
  line L2 (142, 2) -> (142, 12) construction
  line L3 (142, 2) -> (149, 2) construction
  line L4 (145.5, 2) -> (149, 4.0207) construction
  line L5 (145.5, 2) -> (142, 4.0207) construction
  line L6 (145.5, 2) -> (149.8012, 2) construction
  line L7 (142, 4.0207) -> (142, 8.0622) construction
  line L8 (142, 8.0622) -> (149, 4.0207) construction
  circle A0 centre (145.5, 6.0415) radius 2.1
  line L9 (130.5, 0) -> (160.5, 0)
  line L10 (160.5, 0) -> (160.5, 12)
  line L11 (160.5, 12) -> (130.5, 12)
  line L12 (130.5, 12) -> (130.5, 0)
  line L13 (149, 2) -> (142, 2)
  dimension "d540" = 150
  dimension "d541" = 150
  dimension "d542" = 4.0415
  dimension "d543" = 4.0415
  dimension "d544" = 4.2
  dimension "d698" = 12
  constraint coincident L1 L4.end
  constraint horizontal L6
  constraint coincident L2 L5.end
  constraint coincident L2 L7.end
  constraint midpoint L8 A0.centre
  constraint coincident L2.start L3.start
  measures "d540" angle of L3 L4
  measures "d541" angle of L5 L6
  measures "d542" distance of L0.start L5.end
  measures "d543" distance of L5.end L7.end
  measures "d544" diameter of A0
  measures "d698" distance of L9.end L10.end
extrude "Extrude36" cut sketch "Sketch29" along normal up to surface contours A0 end surface at (10.9064, 4, -143.2792) on bodies 2 bodies 2
fillet "Fillet30" radius 3 4 edges at (-12.8153, 12, -145.5) (-22.8153, 12, -145.5) (-22.8153, 2, -145.5) (-22.8153, 0, -145.5) on bodies 2
fillet "Fillet30" radius 8 2 edges at (-22.8153, 49, -145.5) (-12.8153, 42, -145.5) on bodies 2
fillet "Fillet30" radius 2 4 edges at (2.1847, 45.5, -130.5) (2.1847, 45.5, -136.5) (2.1847, 45.5, -154.5) (2.1847, 45.5, -160.5) on bodies 2
fillet "Fillet30" radius 5 2 edges at (20.3847, 6, -130.5) (20.3847, 6, -160.5) on bodies 2
fillet "Fillet30" radius 2 6 edges at (-87.8153, 2, -156.9712) (-87.8153, 2, -134.0288) (-87.8153, -18, -137.0515) (-87.8153, -14, -139.8523) (-87.8153, -14, -151.1477) (-87.8153, -18, -153.9485) on bodies 2
fillet "Fillet30" radius 2 4 edges at (-26.8153, 7, -147.5) (-26.8153, 7, -143.5) (-77.8153, 7, -147.5) (-77.8153, 7, -143.5) on bodies 2
fillet "Fillet30" radius 3 4 edges at (-97.8153, 12, -156.75) (-97.8153, 12, -134.25) (-97.8153, 2, -134.25) (-97.8153, 2, -156.75) on bodies 2
copy_body "Body->Comp6" bodies 1 removing the originals makes body 4 in component "Mount Slide"
copy_body "Body->Comp7" bodies 2 removing the originals makes body 5 in component "Mount Pen"
component "Mount Slide" placed x (1, 0, 0) y (0, 1, 0) z (0, 0, 1) at (0, 0, 0)
component "Mount Pen" placed x (1, 0, 0) y (0, 1, 0) z (0, 0, 1) at (144.9741, 96.9, 114.5105)
equation "l_mount = 18 mm" comment "Distance mounting screws length-wise"
equation "w_mount = 24 mm"
equation "d24 = d25"
equation "d25 = l_mount"
equation "d27 = d26"
equation "d28 = d26"
equation "d29 = d26"
equation "d30 = d22 / 2"
equation "d35 = d_slider_thread + dia_threadnut / 2"
equation "dia_threadnut_shaft = 10.2 mm"
equation "dia_threadnut = 22 mm"
equation "dia_threadnut_screws = 16 mm"
equation "d40 = dia_threadnut_shaft + 0.2 mm"
equation "d41 = dia_threadnut + 0.2 mm"
equation "d47 = ( d48 - d46 ) / 2"
equation "d50 = d49"
equation "d51 = d49"
equation "d52 = d49"
equation "d60 = dia_threadnut_screws"
equation "d62 = d61"
equation "d63 = d61"
equation "d64 = d61"
equation "d66 = d_slider_thread"
equation "d_slider_thread = 30 mm"
equation "height_slider2bottommount = 60 mm"
equation "lever = 100 mm"
equation "d77 = d78"
equation "d81 = hinge_bearing_outerdia + 0.2 mm"
equation "hinge_bearing_outerdia = 10 mm"
equation "hinge_bearing_innerdia = 5 mm"
equation "d84 = d81 + 6 mm"
equation "d85 = d84"
equation "d86 = d84 / 2 + 0.2 mm"
equation "d91 = d90"
equation "d92 = d79 / 2"
equation "d93 = d80 / 2"
equation "d94 = d78 / 2"
equation "d95 = d77 / 2"
equation "hinge_bearring_width = 4 mm"
equation "d100 = hinge_bearing_innerdia + 0.2 mm"
equation "d102 = hinge_bearring_width + 0.2 mm"
equation "d110 = -hinge_bearring_width + 0.2 mm"
equation "d117 = d80"
equation "d118 = d79"
equation "d119 = d120"
equation "d120 = 10.00 mm"
equation "d121 = d120"
equation "d124 = d121 + d78"
equation "d126 = d125"
equation "d134 = d133"
equation "dia_pen = 18 mm"
equation "d168 = dia_pen"
equation "d171 = d169 / 2"
equation "d172 = d168 / 2 + 3 mm"
equation "d175 = d181"
equation "d176 = d175 / 2"
equation "d177 = d176"
equation "d181 = d681"
equation "d188 = d187"